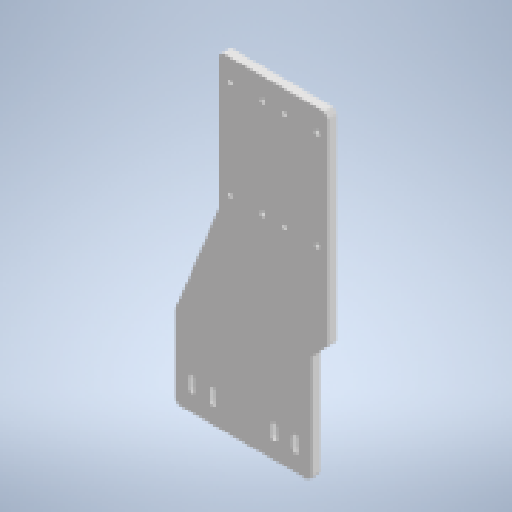
# Autodesk Inventor part: PA1
Saved by Autodesk Inventor 2023 (Build 270158000, 158)
## iProperties
Created: 2025-03-27
Part Number: PA1
Material: Generic
Document SubType Name: Modeling
Designer: huyqu
Density: 1 g/cm^3
Appearance: Default
Mass: 2103.5 g
Surface Area: 3201.69 cm^2
Volume: 2103.5 cm^3
Author: huyqu
Autodesk Inventor part; units mm, degrees
ref_plane "YZ Plane" through (0, 0, 0) normal (1, 0, 0) x (0, 1, 0)
ref_plane "XZ Plane" through (0, 0, 0) normal (0, 1, 0) x (-1, 0, 0)
ref_plane "XY Plane" through (0, 0, 0) normal (0, 0, 1) x (1, 0, 0)
sketch "Sketch1" plane through (0, 0, 0) normal (0, 0, 1) x (1, 0, 0)
  line L0 (0, 0) -> (250, 0)
  line L1 (250, 0) -> (250, 150)
  line L2 (0, 150) -> (0, 0)
  line L3 (0, 150) -> (80, 350)
  line L4 (80, 350) -> (80, 600)
  line L5 (280, 600) -> (280, 230)
  line L6 (250, 150) -> (250, 200)
  line L7 (250, 200) -> (280, 230)
  line L8 (80, 600) -> (280, 600)
  dimension "d0" = 250
  dimension "d1" = 150
  dimension "d3" = 80
  dimension "d5" = 30
  dimension "d6" = 50
  dimension "d8" = 600
  dimension "d9" = 200
  dimension "d10" = 30
  dimension "d11" = 150
  constraints: 18 end point, 3 vertical, 2 horizontal, 1 parallel, 1 perpendicular
  measures "d0" distance of L0.start L0.end
  measures "d1" distance of L0.end L1.end
  measures "d3" distance between parallel lines of L2 L4
  measures "d5" distance between parallel lines of L5 L1
  measures "d6" distance of L1.end L6.end
  measures "d8" distance between parallel lines of L0 L8
  measures "d9" vertical distance of L2.start L3.end
  measures "d10" horizontal distance of L5.end L6.end
  measures "d11" distance of L2.start L0.start
extrude "Extrusion1" add sketch "Sketch1" along normal blind 16
fillet "Fillet1" radius 10 4 edges at (80, 600, 8) (280, 600, 8) (0, 0, 8) (250, 0, 8)
sketch "Sketch9" plane through (0, 0, 16) normal (0, 0, 1) x (1, 0, 0)
  line L0 (0, 150) -> (0, 10) projected
  line L1 (0, 35) -> (250, 35)
  line L2 (250, 10) -> (250, 200) projected
  line L3 (10, 0) -> (240, 0) projected
  circle A0 centre (30, 35) radius 5
  circle A1 centre (69, 35) radius 5
  circle A2 centre (181, 35) radius 5
  circle A3 centre (220, 35) radius 5
  line L4 (25, 35) -> (25, 55)
  line L5 (35, 35) -> (35, 55)
  circle A4 centre (30, 55) radius 5
  circle A5 centre (69, 55) radius 5
  line L6 (64, 55) -> (64, 35)
  line L7 (74, 55) -> (74, 35)
  line L8 (0, 100) -> (250, 100)
  circle A6 centre (125, 50) radius 5
  circle A7 centre (220, 55) radius 5
  line L9 (215, 55) -> (215, 35)
  line L10 (225, 55) -> (225, 35)
  circle A8 centre (181, 55) radius 5
  line L11 (176, 55) -> (176, 35)
  line L12 (186, 55) -> (186, 35)
  point P0 (0, 0)
  point P1 (0, 148.0742)
  point P2 (250, 196.6667)
  point P3 (125, 100)
  dimension "d111" = 35
  dimension "d112" = 30
  dimension "d113" = 10
  dimension "d114" = 20
  dimension "d116" = 10
  dimension "d117" = 10
  dimension "d118" = 10
  dimension "d119" = 20
  dimension "d120" = 100
  dimension "d121" = 10
  dimension "d122" = 50
  dimension "d123" = 30
  dimension "d124" = 20
  dimension "d127" = 29
  dimension "d128" = 29
  dimension "d129" = 20
  dimension "d153" = 10
  dimension "d154" = 0
  dimension "d155" = 10
  dimension "d156" = 10
  dimension "d157" = 10
  constraints: 18 end point, 16 point on circle, 9 centre point, 4 point on line, 2 tangent, 2 vertical, 1 horizontal, 1 midpoint, 15 other
  measures "d112" distance from line of A0.centre L0
  measures "d113" diameter of A0
  measures "d114" distance of L4.start L4.end
  measures "d116" diameter of A1
  measures "d117" diameter of A2
  measures "d118" diameter of A3
  measures "d119" distance of L6.start L6.end
  measures "d120" distance between parallel lines of L3 L8
  measures "d121" diameter of A6
  measures "d122" distance of point (125, 100) A6.centre
  measures "d123" distance from line of L2 A3.centre
  measures "d124" distance of L9.start L9.end
  measures "d127" distance between parallel lines of L9 L12
  measures "d128" distance between parallel lines of L6 L5
  measures "d153" diameter of A7
  measures "d154" horizontal distance of A3.centre A7.centre
  measures "d155" diameter of A8
  measures "d156" diameter of A5
  measures "d157" diameter of A4
extrude "Extrusion7" cut sketch "Sketch9" against normal through all contours A0 L1 | L4 A4 L5 A0 | L1 A0 | A4 | A3 L1 | L1 A3 | A3 L9 A7 L10 | A1 L1 | L6 A5 L7 A1 | L1 A1 | A7 | A5 | A2 L1 | L1 A2 | A2 L11 A8 L12 | A8
sketch "Sketch10" plane through (0, 0, 0) normal (0, 0, -1) x (-1, 0, 0)
  line L0 (-280, 230) -> (-280, 590) projected
  line L1 (-280, 560) -> (-80, 560)
  line L2 (-80, 590) -> (-80, 350) projected
  line L3 (-270, 600) -> (-90, 600) projected
  line L4 (-270, 600) -> (-90, 600) projected
  line L5 (-180, 600) -> (-180, 520)
  line L6 (-200, 580) -> (-160, 580)
  line L7 (-160, 580) -> (-160, 540)
  line L8 (-160, 540) -> (-200, 540)
  line L9 (-200, 540) -> (-200, 580)
  line L10 (-200, 580) -> (-160, 540) construction
  line L11 (-160, 580) -> (-200, 540) construction
  circle A0 centre (-200, 560) radius 4.5
  circle A1 centre (-160, 560) radius 4.5
  circle A2 centre (-260, 560) radius 4.5
  circle A3 centre (-100, 560) radius 4.5
  line L12 (-180, 520) -> (-180, 380)
  line L13 (-200, 400) -> (-160, 400)
  line L14 (-160, 400) -> (-160, 360)
  line L15 (-160, 360) -> (-200, 360)
  line L16 (-200, 360) -> (-200, 400)
  line L17 (-200, 400) -> (-160, 360) construction
  line L18 (-160, 400) -> (-200, 360) construction
  line L19 (-280, 380) -> (-80, 380)
  circle A4 centre (-260, 380) radius 4.5
  circle A5 centre (-100, 380) radius 4.5
  circle A6 centre (-200, 380) radius 4.5
  circle A7 centre (-160, 380) radius 4.5
  point P0 (0, 0)
  point P1 (-280, 243.3333)
  point P2 (-80, 351.9258)
  point P3 (-180, 560)
  dimension "d130" = 40
  dimension "d131" = 80
  dimension "d132" = 40
  dimension "d133" = 40
  dimension "d134" = 9
  dimension "d135" = 9
  dimension "d136" = 9
  dimension "d137" = 9
  dimension "d138" = 60
  dimension "d139" = 60
  dimension "d140" = 140
  dimension "d141" = 40
  dimension "d142" = 40
  dimension "d143" = 9
  dimension "d144" = 220
  dimension "d145" = 9
  dimension "d146" = 9
  dimension "d147" = 9
  dimension "d148" = 60
  dimension "d149" = 60
  constraints: 32 end point, 10 midpoint, 10 point on line, 8 centre point, 4 parallel, 3 horizontal, 3 perpendicular, 2 vertical
  measures "d130" distance between parallel lines of L3 L1
  measures "d131" distance of L5.start L5.end
  measures "d132" distance of L8.end L6.start
  measures "d133" distance of L6.start L6.end
  measures "d134" diameter of A0
  measures "d135" diameter of A1
  measures "d136" diameter of A2
  measures "d137" diameter of A3
  measures "d138" distance from line of L9 A2.centre
  measures "d139" distance from line of A3.centre L7
  measures "d140" distance of L5.end L12.end
  measures "d141" distance of L13.start L13.end
  measures "d142" distance of L13.end L14.end
  measures "d143" diameter of A4
  measures "d144" distance between parallel lines of L19 L3
  measures "d145" diameter of A5
  measures "d146" diameter of A6
  measures "d147" diameter of A7
  measures "d148" distance from line of L16 A4.centre
  measures "d149" distance from line of A5.centre L14
extrude "Extrusion8" cut sketch "Sketch10" against normal through all contours A4 L19 | L19 A4 | A2 L1 | L1 A2 | A6 L16 L19 | L19 L16 A6 | A0 L9 L1 | L1 L9 A0 | L19 A6 L16 | L16 A6 L19 | L9 A0 L1 | L1 A0 L9 | A7 L14 L19 | L19 L14 A7 | L14 L19 A7 | A1 L7 L1 | L1 L7 A1 | L14 A7 L19 | L7 A1 L1 | L1 A1 L7 | A5 L19 | L19 A5 | A3 L1 | L1 A3
fillet "Fillet3" radius 5 4 edges at (280, 230, 8) (250, 200, 8) (0, 150, 8) (80, 350, 8)
body "Solid1"
